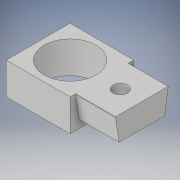
# Autodesk Inventor part: HopperFinal3
Saved by Autodesk Inventor 2018 (Build 220112000, 112)
## iProperties
Created: 2019-03-21
Part Number: HopperFinal3
Material: Generic
Document SubType Name: Modeling
Designer: 871357
Density: 1 g/cm^3
Appearance: Default
Author: 871357
Autodesk Inventor part; units mm, degrees
ref_plane "YZ Plane" through (0, 0, 0) normal (1, 0, 0) x (0, 1, 0)
ref_plane "XZ Plane" through (0, 0, 0) normal (0, 1, 0) x (-1, 0, 0)
ref_plane "XY Plane" through (0, 0, 0) normal (0, 0, 1) x (1, 0, 0)
sketch "Sketch1" plane through (0, 0, 0) normal (0, 1, 0) x (-1, 0, 0)
  line L0 (-10.16, 10.16) -> (10.16, 10.16)
  line L1 (10.16, 10.16) -> (10.16, -10.16)
  line L2 (10.16, -10.16) -> (-10.16, -10.16)
  line L3 (-10.16, -10.16) -> (-10.16, 10.16)
  circle A0 centre (0, 0) radius 8.255
  dimension "d0" = 20.32
  dimension "d1" = 20.32
  dimension "d2" = 10.16
  dimension "d3" = 10.16
  dimension "d4" = 16.51
  constraints: 8 end point, 2 parallel, 1 centre point, 1 coincident, 1 horizontal, 1 perpendicular
  measures "d0" distance between parallel lines of L3 L1
  measures "d1" distance between parallel lines of L2 L0
  measures "d2" distance from line of L2 point (0, 0)
  measures "d3" distance from line of point (0, 0) L1
  measures "d4" diameter of A0
extrude "Extrusion1" add sketch "Sketch1" along normal blind 12.7
sketch "Sketch2" plane through (10.16, 0, 10.16) normal (1, 0, 0) x (0, 0, -1)
  line L0 (1.778, 12.446) -> (2.921, 5.08)
  line L1 (2.921, 5.08) -> (17.399, 5.08)
  line L2 (17.399, 5.08) -> (18.542, 12.446)
  line L3 (18.542, 12.446) -> (1.778, 12.446)
  line L4 (20.32, 0) -> (0, 0) projected
  line L5 (20.32, 0) -> (20.32, 12.7) projected
  point P0 (10.16, 0)
  dimension "d7" = 16.764
  dimension "d8" = 14.478
  dimension "d9" = 7.366
  dimension "d10" = 5.08
  dimension "d11" = 2.921
  constraints: 8 end point, 1 equal length, 1 horizontal, 1 parallel
  measures "d7" distance of L2.end L0.start
  measures "d8" distance of L0.end L1.end
  measures "d9" distance between parallel lines of L1 L3
  measures "d10" distance between parallel lines of L4 L1
  measures "d11" distance from line of L5 L1.end
extrude "Extrusion2" add sketch "Sketch2" along normal blind 12.7
sketch "Sketch3" plane through (10.16, 12.446, 8.382) normal (0, 1, 0) x (1, 0, 0)
  circle A0 centre (5.842, 8.382) radius 2.286
  line L0 (12.7, 16.764) -> (12.7, 0) projected
  point P0 (-10.16, 8.382)
  dimension "d14" = 4.572
  dimension "d15" = 6.858
  constraints: 1 centre point
  measures "d14" diameter of A0
  measures "d15" distance from line of L0 A0.centre
extrude "Extrusion3" cut sketch "Sketch3" against normal blind 17.78
sketch "Sketch4" plane through (10.16, 12.446, 8.382) normal (0, 1, 0) x (1, 0, 0)
  circle A0 centre (5.842, 8.382) radius 2.286 projected
  line L0 (0, 0) -> (0, 16.764) projected
  line L1 (0, 0) -> (12.7, 0) projected
  line L2 (12.7, 16.764) -> (12.7, 0) projected
  line L3 (0, 16.764) -> (12.7, 16.764) projected
  point P0 (-10.16, 8.382)
extrude "Extrusion4" add sketch "Sketch4" along normal up to surface (0.254 mm away)
sketch "Sketch5" plane through (0, 0, 0) normal (0, -1, 0) x (1, 0, 0)
  line L0 (14.2823, 20.4865) -> (-14.5737, 20.4865)
  line L1 (-14.5737, 20.4865) -> (-14.5737, -26.9822)
  line L2 (-14.5737, -26.9822) -> (14.2823, -26.9822)
  line L3 (14.2823, -26.9822) -> (14.2823, 20.4865)
  point P0 (0, 0)
  constraints: 8 end point, 2 parallel, 1 horizontal, 1 perpendicular
extrude "Extrusion5" cut sketch "Sketch5" against normal blind 2.54
body "Solid1"
